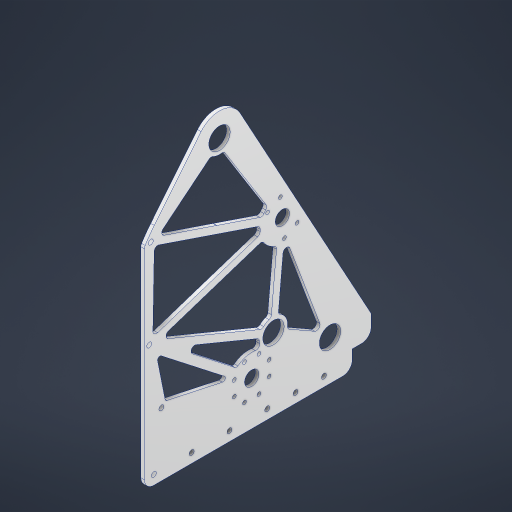
# Autodesk Inventor part: CORL_001_MainPlate
Saved by Autodesk Inventor 2024.2 (Build 282272000, 272)
## iProperties
Created: 2024-08-01
Part Number: CORL_001_MainPlate
Material: Aluminum 6061
Document SubType Name: Modeling
Designer: Bryan
Density: 2.7 g/cm^3
Appearance: Aluminum - Flat
Mass: 689.904 g
Surface Area: 1304.9 cm^2
Volume: 255.52 cm^3
Author: Bryan
Autodesk Inventor part; units mm, degrees
ref_plane "YZ Plane" through (0, 0, 0) normal (1, 0, 0) x (0, 1, 0)
ref_plane "XZ Plane" through (0, 0, 0) normal (0, 1, 0) x (-1, 0, 0)
ref_plane "XY Plane" through (0, 0, 0) normal (0, 0, 1) x (1, 0, 0)
sketch "Sketch1" plane through (0, 0, 0) normal (1, 0, 0) x (0, 1, 0)
  line L0 (0, 0) -> (0, -205.0034) construction
  circle A0 centre (0, 0) radius 25.4 construction
  circle A1 centre (0, -205.0034) radius 25.4 construction
  circle A2 centre (0, 0) radius 14.2875 construction
  circle A3 centre (0, -205.0034) radius 14.2875
  line L1 (0, -266.7) -> (406.4, -266.7) construction
  line L2 (0, 0) -> (0, 69.85) construction
  line L3 (0, 69.85) -> (406.4, 69.85) construction
  line L4 (-25.4, 0) -> (-25.4, -205.0034) construction
  arc A4 (-25.4, 0) -> (-25.4, 0) centre (0, 0) ccw construction
  arc A5 (-25.4, -205.0034) -> (0, -230.4034) centre (0, -205.0034) ccw construction
  line L5 (-53.975, 44.45) -> (-28.575, 44.45)
  line L6 (-28.575, 44.45) -> (-28.575, -234.95) construction
  line L7 (-28.575, -234.95) -> (-53.975, -234.95)
  line L8 (-53.975, -234.95) -> (-53.975, 44.45)
  line L9 (-28.575, -234.95) -> (-28.575, -260.35)
  circle A6 centre (-41.275, 44.45) radius 3.2512 construction
  circle A7 centre (-41.275, 31.75) radius 3.2512
  circle A8 centre (-41.275, 19.05) radius 3.2512 construction
  circle A9 centre (-41.275, 6.35) radius 3.2512 construction
  circle A10 centre (-41.275, -6.35) radius 3.2512 construction
  circle A11 centre (-41.275, -19.05) radius 3.2512
  circle A12 centre (-41.275, -31.75) radius 3.2512 construction
  circle A13 centre (-41.275, -44.45) radius 3.2512 construction
  circle A14 centre (-41.275, -57.15) radius 3.2512 construction
  circle A15 centre (-41.275, -69.85) radius 3.2512
  circle A16 centre (-41.275, -82.55) radius 3.2512 construction
  circle A17 centre (-41.275, -95.25) radius 3.2512 construction
  circle A18 centre (-41.275, -107.95) radius 3.2512 construction
  circle A19 centre (-41.275, -120.65) radius 3.2512
  circle A20 centre (-41.275, -133.35) radius 3.2512 construction
  circle A21 centre (-41.275, -146.05) radius 3.2512 construction
  circle A22 centre (-41.275, -158.75) radius 3.2512
  circle A23 centre (-41.275, -171.45) radius 3.2512 construction
  circle A24 centre (-41.275, -184.15) radius 3.2512 construction
  circle A25 centre (-41.275, -196.85) radius 3.2512
  circle A26 centre (-41.275, -209.55) radius 3.2512 construction
  circle A27 centre (-41.275, -222.25) radius 3.2512 construction
  circle A28 centre (-41.275, -234.95) radius 3.2512 construction
  line L10 (0, -205.0034) -> (142.7545, -151.6469) construction
  circle A29 centre (171.3054, -140.9756) radius 30.48 construction
  circle A30 centre (171.3054, -140.9756) radius 9.525
  circle A31 centre (171.3054, -140.9756) radius 30 construction
  circle A32 centre (155.3994, -160.7786) radius 2.4892
  circle A33 centre (146.0553, -143.7312) radius 2.4892
  circle A34 centre (196.5555, -138.2201) radius 2.4892
  circle A35 centre (187.2114, -121.1727) radius 2.4892
  line L11 (196.5555, -138.2201) -> (187.2114, -121.1727) construction
  line L12 (187.2114, -121.1727) -> (146.0553, -143.7312) construction
  line L13 (146.0553, -143.7312) -> (155.3994, -160.7786) construction
  line L14 (155.3994, -160.7786) -> (196.5555, -138.2201) construction
  circle A36 centre (171.3054, -140.9756) radius 25.4 construction
  line L15 (0, 0) -> (249.8384, -215.9) construction
  circle A37 centre (305.9915, -56.4229) radius 25.4 construction
  arc A38 (305.9915, -56.4229) -> (0, 0) centre (139.099, -103.5757) ccw construction
  line L16 (0, -205.0034) -> (59.0925, -345.4806) construction
  line L17 (59.0925, -345.4806) -> (281.6851, -514.35) construction
  circle A39 centre (281.6851, -514.35) radius 50.8 construction
  line L18 (294.3851, -565.15) -> (268.9851, -565.15) construction
  circle A40 centre (59.0925, -345.4806) radius 50.8 construction
  circle A41 centre (0, -205.0034) radius 152.4 construction
  line L19 (0, -205.0034) -> (152.0099, -215.9) construction
  line L20 (152.0099, -215.9) -> (403.3467, -93.8582) construction
  circle A42 centre (403.3467, -93.8582) radius 50.8 construction
  circle A43 centre (152.0099, -215.9) radius 50.8 construction
  line L21 (305.9915, -56.4229) -> (231.2092, 35.8159) construction
  circle A44 centre (231.2092, 35.8159) radius 6.35 construction
  circle A45 centre (231.2092, 35.8159) radius 3.2512
  circle A46 centre (305.9915, -56.4229) radius 14.2875
  circle A47 centre (403.3467, -93.8582) radius 25.4 construction
  circle A48 centre (152.0099, -215.9) radius 25.4 construction
  line L22 (392.252, -71.0094) -> (140.9152, -193.0512) construction
  line L23 (163.1047, -238.7488) -> (414.4414, -116.707) construction
  circle A49 centre (305.9915, -56.4229) radius 31.75 construction
  circle A50 centre (59.0925, -345.4806) radius 25.4 construction
  line L24 (0, -205.0034) -> (80.5364, -331.8675) construction
  circle A51 centre (112.4851, 38.0456) radius 6.35 construction
  circle A52 centre (112.4851, 38.0456) radius 3.2512
  line L25 (231.2092, 35.8159) -> (112.4851, 38.0456) construction
  line L26 (112.4851, 38.0456) -> (0, 0) construction
  line L27 (-28.575, 44.45) -> (110.7715, 67.5208)
  line L28 (248.2424, 31.1989) -> (325.973, -31.749)
  arc A53 (248.2424, 31.1989) -> (110.7715, 67.5208) centre (139.099, -103.5757) ccw
  line L29 (-28.575, -260.35) -> (0, -260.35)
  arc A54 (321.2522, -84.2648) -> (325.973, -31.749) centre (305.9915, -56.4229) ccw
  line L30 (321.2522, -84.2648) -> (0, -260.35)
  circle A55 centre (4.9608, -99.7986) radius 9.6012
  circle A56 centre (4.9608, -99.7986) radius 25.4 construction
  circle A57 centre (4.9608, -99.7986) radius 30 construction
  circle A58 centre (43.377, -129.0086) radius 14.2875
  circle A59 centre (28.4274, -90.0784) radius 2.4892
  circle A60 centre (14.681, -76.3321) radius 2.4892
  circle A61 centre (-4.7593, -76.3321) radius 2.4892
  circle A62 centre (-18.5057, -90.0784) radius 2.4892
  circle A63 centre (-18.5057, -109.5188) radius 2.4892
  circle A64 centre (-4.7593, -123.2651) radius 2.4892
  circle A65 centre (14.681, -123.2651) radius 2.4892
  circle A66 centre (28.4274, -109.5188) radius 2.4892
  line L31 (-18.5057, -90.0784) -> (-18.5057, -109.5188) construction
  circle A67 centre (43.377, -129.0086) radius 38.1 construction
  circle A68 centre (4.9608, -99.7986) radius 10.16 construction
  point P0 (-41.275, 44.45)
  point P1 (281.6851, -565.15)
  dimension "d165" = 50.8
  dimension "d217" = 50.8
  dimension "d0" = 205.0034
  dimension "d1" = 50.8
  dimension "d3" = 28.575
  dimension "d4" = 28.575
  dimension "d15" = 69.85
  dimension "d19" = 25.4
  dimension "d21" = 3.175
  dimension "d22" = 44.45
  dimension "d23" = 6.5024
  dimension "d27" = 12.7
  dimension "d68" = 60.96
  dimension "d73" = 152.4
  dimension "d74" = 19.05
  dimension "d93" = 60
  dimension "d130" = 4.9784
  dimension "d132" = 50.8
  dimension "d133" = 279.4
  dimension "d139" = 25.4
  dimension "d144" = 6.35
  dimension "d145" = 406.4
  dimension "d147" = 330.2
  dimension "d148" = 50.8
  dimension "d149" = 311.15
  dimension "d151" = 50.8
  dimension "d152" = 279.4
  dimension "d153" = 101.6
  dimension "d154" = 304.8
  dimension "d155" = 150
  dimension "d156" = 150
  dimension "d157" = 12.7
  dimension "d158" = 6.5024
  dimension "d161" = 340.1572
  dimension "d162" = 50.8
  dimension "d163" = 50.8
  dimension "d164" = 63.5
  dimension "d166" = 12.7
  dimension "d167" = 6.5024
  dimension "d168" = 9.594
  dimension "d170" = 24.594
  dimension "d186" = 19.4403
  dimension "d215" = 76.2
  dimension "d216" = 19.2024
  dimension "d218" = 60
  dimension "d219" = 28.575
  dimension "d221" = 4.9784
  dimension "d224" = 360
  dimension "d247" = 87.503
  dimension "d256" = 76.2
  dimension "d257" = 20.32
  dimension "d258" = 304.1396
  dimension "d266" = 29.21
  dimension "d268" = 118.745
  constraints: 66 centre point, 65 end point, 29 coincident, 25 point on circle, 16 tangent, 10 equal radius, 7 equal length, 7 vertical, 6 horizontal, 4 parallel, 4 vertical alignment, 3 midpoint, 1 concentric, 1 perpendicular, 1 point on line, 72 other
  measures "d0" distance of L0.start L0.end
  measures "d1" diameter of A0
  measures "d3" diameter of A2
  measures "d4" diameter of A3
  measures "d15" distance of L2.start L2.end
  measures "d19" distance of L5.start L5.end
  measures "d21" distance between parallel lines of L4 L6
  measures "d22" distance from line of L5 L0.start
  measures "d23" diameter of A6
  measures "d27" distance of A6.centre A7.centre
  measures "d68" diameter of A29
  measures "d73" distance of L0.end L10.end
  measures "d74" diameter of A30
  measures "d93" diameter of A31
  measures "d130" diameter of A32
  measures "d132" diameter of A36
  measures "d133" distance between parallel lines of L5 L7
  measures "d139" distance of L6.end L9.end
  measures "d144" vertical distance of L9.end L1.start
  measures "d145" distance of L2.end L3.end
  measures "d147" distance of L0.start L15.end
  measures "d148" diameter of A37
  measures "d149" distance of L0.start L21.start
  measures "d151" vertical distance of L1.end L15.end
  measures "d152" distance of L16.end L17.end
  measures "d153" diameter of A39
  measures "d154" distance from line of L9.end L18
  measures "d155" angle of L17 L16
  measures "d156" angle of L19 L20
  measures "d157" diameter of A44
  measures "d158" diameter of A45
  measures "d161" distance of L0.end A46.centre
  measures "d162" diameter of A47
  measures "d163" diameter of A48
  measures "d164" diameter of A49
  measures "d166" diameter of A51
  measures "d167" diameter of A52
  measures "d168" angle of L16 L24
  measures "d170" angle of L19 L10
  measures "d186" distance of L12.end L13.end
  measures "d215" distance from line of L21.start L20
  measures "d216" diameter of A55
  measures "d218" diameter of A57
  measures "d219" diameter of A58
  measures "d221" diameter of A59
  measures "d247" distance of L0.end A58.centre
  measures "d256" diameter of A67
  measures "d257" diameter of A68
  measures "d258" distance of A55.centre L21.start
  measures "d266" vertical distance of A55.centre A58.centre
  measures "d268" distance of L25.start L25.end
extrude "Extrusion1" add sketch "Sketch1" along normal blind 4.7625
fillet "Fillet2" radius 12.7 3 edges at (2.3813, -53.975, 44.45) (2.3813, -53.975, -234.95) (2.3813, -28.575, -260.35)
sketch "Sketch5" plane through (4.7625, 0, 0) normal (1, 0, 0) x (0, 0, -1)
  circle A0 centre (-35.8159, 231.2092) radius 6.35
  circle A1 centre (-38.0456, 112.4851) radius 6.35
  line L0 (-38.1, -28.0529) -> (-64.4683, 131.2102)
  arc A2 (-52.8092, 211.4673) -> (-64.4683, 131.2102) centre (117.2224, 145.7909) ccw
  line L1 (-52.8092, 211.4673) -> (36.6838, 321.9767)
  arc A3 (78.6964, 318.2001) -> (36.6838, 321.9767) centre (56.4229, 305.9915) ccw
  line L2 (78.6964, 318.2001) -> (254, -1.6262)
  line L3 (254, -1.6262) -> (254, -15.875)
  arc A4 (247.65, -22.225) -> (254, -15.875) centre (247.65, -15.875) ccw
  line L4 (247.65, -22.225) -> (228.6, -22.225)
  line L5 (228.6, -22.225) -> (228.6, -41.275)
  arc A5 (222.25, -47.625) -> (228.6, -41.275) centre (222.25, -41.275) ccw
  line L6 (222.25, -47.625) -> (-31.75, -47.625)
  arc A6 (-38.1, -41.275) -> (-31.75, -47.625) centre (-31.75, -41.275) ccw
  line L7 (-38.1, -41.275) -> (-38.1, -28.0529)
  circle A7 centre (205.0034, 0) radius 19.05
  circle A8 centre (140.9756, 171.3054) radius 30
  circle A9 centre (56.4229, 305.9915) radius 19.05
  line L8 (56.4229, 305.9915) -> (-35.8159, 231.2092)
  line L9 (-35.8159, 231.2092) -> (-38.0456, 112.4851)
  line L10 (129.0086, 43.377) -> (205.0034, 0)
  line L11 (205.0034, 0) -> (140.9756, 171.3054)
  line L12 (140.9756, 171.3054) -> (56.4229, 305.9915)
  line L13 (-31.0958, 228.9049) -> (55.2471, 298.9071)
  line L14 (55.2471, 298.9071) -> (136.6843, 169.1839)
  line L15 (136.6843, 169.1839) -> (195.9348, 10.66)
  line L16 (195.9348, 10.66) -> (115.3502, 56.6568)
  line L17 (-33.158, 119.104) -> (-31.0958, 228.9049)
  line L18 (-35.8159, 231.2092) -> (140.9756, 171.3054)
  line L19 (140.9756, 171.3054) -> (-38.0456, 112.4851)
  line L20 (-38.0456, 112.4851) -> (129.0086, 43.377)
  line L21 (140.9756, 171.3054) -> (129.0086, 43.377)
  line L22 (-43.616, 109.6356) -> (110.1438, 46.0272)
  line L23 (-37.0067, 117.2093) -> (113.7849, 54.8288)
  line L24 (166.2301, 174.5902) -> (-35.0095, 108.4697)
  line L25 (163.2569, 183.6392) -> (-37.9827, 117.5188)
  line L26 (-39.9815, 227.5922) -> (128.8822, 170.3747)
  line L27 (-36.3152, 236.4069) -> (132.5484, 179.1893)
  line L28 (136.8754, 178.6072) -> (122.5489, 25.4557)
  line L29 (146.1797, 175.8036) -> (133.5494, 40.7852)
  line L30 (-36.9307, 171.8472) -> (51.465, 141.8953)
  line L31 (51.465, 141.8953) -> (52.5799, 201.2573)
  line L32 (-36.9307, 171.8472) -> (52.5799, 201.2573)
  line L33 (47.6922, 194.6384) -> (46.8256, 148.4957)
  line L34 (46.8256, 148.4957) -> (-21.8852, 171.7776)
  line L35 (-21.8852, 171.7776) -> (47.6922, 194.6384)
  line L36 (57.4675, 207.8762) -> (56.1044, 135.2948)
  line L37 (56.1044, 135.2948) -> (-51.9763, 171.9167)
  line L38 (-51.9763, 171.9167) -> (57.4675, 207.8762)
  line L39 (51.465, 141.8953) -> (45.4815, 77.9311)
  line L40 (45.4815, 77.9311) -> (134.9921, 107.3412)
  line L41 (51.465, 141.8953) -> (134.9921, 107.3412)
  line L42 (121.2947, 107.8537) -> (50.9003, 84.7245)
  line L43 (50.9003, 84.7245) -> (55.6059, 135.0283)
  line L44 (55.6059, 135.0283) -> (121.2947, 107.8537)
  line L45 (148.6895, 106.8287) -> (40.0627, 71.1377)
  line L46 (40.0627, 71.1377) -> (47.3241, 148.7623)
  line L47 (47.3241, 148.7623) -> (148.6895, 106.8287)
  line L48 (52.5799, 201.2573) -> (56.4229, 305.9915)
  line L49 (48.055, 207.819) -> (51.2959, 296.1452)
  line L50 (57.4693, 204.629) -> (60.8161, 295.839)
  arc A10 (247.65, -28.575) -> (260.35, -15.875) centre (247.65, -15.875) ccw projected
  line L51 (260.35, -15.875) -> (260.35, 0) projected
  line L52 (260.35, 0) -> (84.2648, 321.2522) projected
  arc A11 (84.2648, 321.2522) -> (31.749, 325.973) centre (56.4229, 305.9915) ccw projected
  line L53 (31.749, 325.973) -> (-31.1989, 248.2424) projected
  arc A12 (-31.1989, 248.2424) -> (-67.5208, 110.7715) centre (103.5757, 139.099) ccw projected
  line L54 (-67.5208, 110.7715) -> (-44.45, -28.575) projected
  line L55 (-44.45, -28.575) -> (-44.45, -41.275) projected
  arc A13 (-44.45, -41.275) -> (-31.75, -53.975) centre (-31.75, -41.275) ccw projected
  line L56 (-31.75, -53.975) -> (222.25, -53.975) projected
  arc A14 (222.25, -53.975) -> (234.95, -41.275) centre (222.25, -41.275) ccw projected
  line L57 (234.95, -41.275) -> (234.95, -28.575) projected
  line L58 (234.95, -28.575) -> (247.65, -28.575) projected
  circle A15 centre (109.5188, 28.4274) radius 2.4892 projected
  circle A16 centre (123.2651, -4.7593) radius 2.4892 projected
  circle A17 centre (90.0784, -18.5057) radius 2.4892 projected
  circle A18 centre (76.3321, 14.681) radius 2.4892 projected
  circle A19 centre (129.0086, 43.377) radius 14.2875 projected
  circle A20 centre (99.7986, 4.9608) radius 9.6012 projected
  circle A21 centre (196.85, -41.275) radius 3.2512 projected
  circle A22 centre (158.75, -41.275) radius 3.2512 projected
  circle A23 centre (120.65, -41.275) radius 3.2512 projected
  circle A24 centre (69.85, -41.275) radius 3.2512 projected
  circle A25 centre (19.05, -41.275) radius 3.2512 projected
  circle A26 centre (-31.75, -41.275) radius 3.2512 projected
  circle A27 centre (90.0784, 28.4274) radius 2.4892 projected
  circle A28 centre (76.3321, -4.7593) radius 2.4892 projected
  circle A29 centre (109.5188, -18.5057) radius 2.4892 projected
  circle A30 centre (123.2651, 14.681) radius 2.4892 projected
  circle A31 centre (-38.0456, 112.4851) radius 3.2512 projected
  circle A32 centre (56.4229, 305.9915) radius 14.2875 projected
  circle A33 centre (-35.8159, 231.2092) radius 3.2512 projected
  circle A34 centre (121.1727, 187.2114) radius 2.4892 projected
  circle A35 centre (138.2201, 196.5555) radius 2.4892 projected
  circle A36 centre (143.7312, 146.0553) radius 2.4892 projected
  circle A37 centre (160.7786, 155.3994) radius 2.4892 projected
  circle A38 centre (140.9756, 171.3054) radius 9.525 projected
  circle A39 centre (205.0034, 0) radius 14.2875 projected
  circle A40 centre (129.0086, 43.377) radius 19.05
  circle A41 centre (99.7986, 4.9608) radius 30
  line L59 (-38.0456, 112.4851) -> (99.7986, 4.9608)
  line L60 (99.7986, 4.9608) -> (129.0086, 43.377)
  line L61 (-7.4906, 94.691) -> (111.2202, 2.0915)
  line L62 (99.7986, 4.9608) -> (45.4815, 77.9311)
  line L63 (97.3778, 0.237) -> (42.4462, 74.0328)
  line L64 (105.0184, 5.9245) -> (57.8018, 69.3557)
  circle A42 centre (205.0034, 0) radius 14.2875 projected
  line L65 (96.0075, 7.8434) -> (125.2175, 46.2596)
  line L66 (99.7986, 4.9608) -> (205.0034, 0)
  line L67 (100.0229, 9.718) -> (202.5451, 4.8837)
  line L68 (103.5897, 2.0783) -> (132.7997, 40.4945)
  line L69 (126.6477, 39.2409) -> (214.072, -10.66)
  line L70 (214.072, -10.66) -> (145.4367, 172.9728)
  point P0 (0, 0)
  point P1 (142.9587, 141.371)
  point P2 (191.345, 13.2798)
  point P3 (194.0846, 15.6103)
  point P4 (146.8846, 141.8931)
  point P5 (133.4751, 142.2582)
  point P6 (114.3227, 157.5352)
  point P7 (-24.3482, 111.9726)
  point P8 (111.3944, 176.3002)
  point P9 (-31.1765, 224.6087)
  point P10 (-54.5444, 120.5889)
  point P11 (111.3495, 166.5842)
  point P12 (-26.1084, 232.9484)
  point P13 (114.4511, 185.3214)
  point P14 (121.1937, 193.8592)
  point P15 (62.1964, 287.8374)
  point P16 (45.0944, 290.6759)
  point P17 (-32.0431, 178.4661)
  point P18 (37.5344, 201.3268)
  point P19 (36.4195, 141.9648)
  point P20 (-32.2914, 165.2467)
  point P21 (57.2193, 194.6568)
  point P22 (56.3527, 148.5142)
  point P23 (41.3406, 84.7981)
  point P24 (46.0462, 135.1019)
  point P25 (129.5733, 100.5478)
  point P26 (59.1789, 77.4186)
  point P27 (65.1624, 141.3828)
  point P28 (130.8512, 114.2082)
  point P29 (57.5899, 207.9164)
  point P30 (60.5058, 287.3842)
  point P31 (62.7917, 204.659)
  point P32 (53.8187, 207.9057)
  point P33 (50.9872, 287.7334)
  point P34 (129.8235, 180.1127)
  point P35 (60.6149, 290.3566)
  point P36 (51.6549, 146.9706)
  point P37 (51.5611, 147.0095)
  point P38 (51.5598, 146.9394)
  point P39 (52.6031, 206.2779)
  point P40 (57.407, 204.6502)
  point P41 (143.7837, 150.1896)
  point P42 (134.0364, 45.9909)
  point P43 (63.2565, 21.7112)
  point P44 (234.95, -34.925)
  point P45 (125.5214, 57.2324)
  point P46 (57.3578, 26.3886)
  point P47 (53.4598, 29.4795)
  point P48 (125.9847, 62.1855)
  point P49 (119.6707, 54.1907)
  point P50 (135.005, 56.3453)
  point P51 (135.4683, 61.2984)
  point P52 (96.5825, 26.6734)
  point P53 (88.0937, 51.1529)
  point P54 (147.3887, 38.3696)
  point P55 (59.6038, 66.9349)
  point P56 (85.9328, 31.5642)
  point P57 (78.2922, 25.8768)
  point P58 (30.2452, 75.5228)
  point P59 (-48.3709, 98.4476)
  point P60 (79.3732, 26.9336)
  point P61 (43.7757, 136.1322)
  point P62 (43.3258, 136.249)
  point P63 (140.0614, 110.3981)
  point P64 (139.4433, 103.7907)
  point P65 (145.8295, 144.7161)
  point P66 (144.4367, 148.4424)
  point P67 (195.8262, 10.9504)
  point P68 (195.6655, 10.8137)
  point P69 (143.0683, 40.8356)
  point P70 (133.7051, 173.9295)
  point P71 (-37.0246, 166.8505)
  point P72 (-37.9264, 118.834)
  point P73 (-35.5419, 118.3207)
  point P74 (132.5563, 175.7595)
  point P75 (131.6523, 173.2551)
  point P76 (59.5514, 292.0507)
  point P77 (48.9587, 293.8088)
  point P78 (74.9197, 30.4075)
  point P79 (114.373, 31.1827)
  point P80 (121.1704, 26.0143)
  point P81 (52.7661, 206.3315)
  point P82 (52.7621, 206.224)
  point P83 (55.7244, 286.9543)
  point P84 (-31.4417, 234.7555)
  point P85 (41.6252, 293.9943)
  point P86 (-36.836, 176.8913)
  point P87 (-35.8769, 227.9586)
  point P88 (-33.2904, 233.2567)
  point P89 (-23.9775, 101.5114)
  point P90 (76.144, 23.4124)
  dimension "d191" = 12.7
  dimension "d192" = 60
  dimension "d193" = 4.7625
  dimension "d194" = 4.7625
  dimension "d195" = 4.7625
  dimension "d196" = 4.7625
  dimension "d197" = 4.7625
  dimension "d198" = 4.7625
  dimension "d199" = 4.7625
  dimension "d200" = 4.7625
  dimension "d201" = 4.7625
  dimension "d204" = 4.7625
  dimension "d205" = 4.7625
  dimension "d206" = 4.7625
  dimension "d207" = 4.7625
  dimension "d210" = 4.7625
  dimension "d211" = 4.7625
  dimension "d226" = 4.7625
  dimension "d227" = 6.35
  dimension "d228" = 6.35
  dimension "d229" = 6.35
  dimension "d230" = 6.35
  dimension "d231" = 6.35
  dimension "d232" = 6.35
  dimension "d233" = 6.35
  dimension "d234" = 19.05
  dimension "d235" = 6.35
  dimension "d236" = 6.35
  dimension "d237" = 6.35
  dimension "d238" = 4.7625
  dimension "d239" = 4.7625
  dimension "d240" = 4.7625
  dimension "d242" = 6.35
  dimension "d243" = 6.35
  dimension "d244" = 6.35
  dimension "d248" = 4.7625
  dimension "d249" = 60
  dimension "d250" = 4.7625
  dimension "d251" = 4.7625
  dimension "d252" = 4.7625
  dimension "d259" = 4.7625
  dimension "d260" = 4.7625
  dimension "d261" = 4.7625
  dimension "d262" = 4.7625
  constraints: 126 end point, 15 parallel, 14 point on circle, 12 centre point, 8 point on line, 6 midpoint, 5 coincident, 2 concentric, 1 equal radius, 11 other
  measures "d191" diameter of A0
  measures "d192" diameter of A8
  measures "d193" distance between parallel lines of L8 L13
  measures "d194" distance between parallel lines of L20 L22
  measures "d195" distance between parallel lines of L20 L23
  measures "d196" distance between parallel lines of L19 L24
  measures "d197" distance between parallel lines of L19 L25
  measures "d198" distance between parallel lines of L18 L26
  measures "d199" distance between parallel lines of L18 L27
  measures "d200" distance between parallel lines of L21 L28
  measures "d201" distance between parallel lines of L21 L29
  measures "d204" distance between parallel lines of L32 L35
  measures "d205" distance between parallel lines of L32 L38
  measures "d206" distance between parallel lines of L41 L44
  measures "d207" distance between parallel lines of L41 L47
  measures "d210" distance between parallel lines of L48 L49
  measures "d211" distance between parallel lines of L48 L50
  measures "d226" distance between parallel lines of L17 L9
  measures "d228" distance between parallel lines of L56 L6
  measures "d229" distance between parallel lines of L52 L2
  measures "d230" distance from line of point (234.95, -34.925) L5
  measures "d231" distance between parallel lines of L58 L4
  measures "d232" distance between parallel lines of L51 L3
  measures "d233" radius of A4
  measures "d234" distance of L4.end L5.end
  measures "d235" radius of A5
  measures "d236" radial gap between concentric circles of A11 A3
  measures "d237" distance between parallel lines of L53 L1
  measures "d238" radial gap between concentric circles of A9 A32
  measures "d239" radial gap between concentric circles of A39 A7
  measures "d240" radial gap between concentric circles of A19 A40
  measures "d242" distance between parallel lines of L54 L0
  measures "d243" distance between parallel lines of L55 L7
  measures "d244" radius of A6
  measures "d248" distance between parallel lines of L10 L16
  measures "d249" diameter of A41
  measures "d250" distance between parallel lines of L59 L61
  measures "d251" distance between parallel lines of L62 L63
  measures "d252" distance between parallel lines of L62 L64
  measures "d259" distance between parallel lines of L60 L65
  measures "d260" distance between parallel lines of L66 L67
  measures "d261" distance between parallel lines of L60 L68
  measures "d262" distance between parallel lines of L10 L69
extrude "Extrusion5" cut sketch "Sketch5" against normal blind 4.7625 contours L13 A9 L49 L27 | L8 L9 A33 L1 | L49 A9 L48 L38 L27 | L1 A33 | L26 L38 L17 | L26 L32 L17 L38 | A9 L50 L27 L36 L38 L48 | L48 L38 L36 L27 | L31 L47 L46 L25 L30 L17 L32 L26 | L26 L36 L25 L47 L31 | L14 A8 L27 L50 A9 | L26 A8 L25 L36 | L47 L25 L31 | L31 L25 L46 L47 | L30 L25 L37 L17 | L37 L25 L17 | A8 L28 L47 L24 | L47 L28 L41 L24 | L37 L36 L24 L41 L28 L40 L23 L39 | L24 L36 L37 | L39 L23 L46 L24 | L46 L23 L24 | L15 A7 L16 A40 L29 L45 L47 A8 | L22 L46 L45 L63 L61 | L40 L28 L45 L23 | L22 L63 L45 L46 | L63 L45 L22 L62 A41 L61 | L47 L45 L29 | L45 L28 A40 L23 | L22 L45 L63 | L22 L64 A41 L62 | A19 L16 L28 L20 | L20 L28 L65 A19 | A40 L65 A41 L64 L22 | A19 L10 L29 L16 | L28 L16 L21 L20 | L20 L65 L28 | L65 L28 L60 A19 | A40 A41 L65 | L16 L29 L10 L21 | A19 L69 L68 L28 L60 L10 | A19 L68 L69 | L20 L60 L28 L65 | L60 L28 A19 | L33 L34 L35 | L42 L43 L44
fillet "Fillet5" radius 4.7625 23 edges at (2.3813, 224.6087, 31.1765) (2.3813, 232.9484, 26.1084) (2.3813, 290.6759, -45.0944) (2.3813, 287.8374, -62.1964) (2.3813, 193.8592, -121.1937) (2.3813, 185.3214, -114.4511) (2.3813, 176.3002, -111.3944) (2.3813, 166.5842, -111.3495) (2.3813, 157.5352, -114.3227) (2.3813, 142.2582, -133.4751) (2.3813, 141.371, -142.9587) (2.3813, 141.8931, -146.8846) (2.3813, 111.9726, 24.3482) (2.3813, 46.0272, -110.1438) (2.3813, 54.8288, -113.7849) (2.3813, 62.1855, -125.9847) (2.3813, 61.2984, -135.4683) (2.3813, 38.3696, -147.3887) (2.3813, 15.6103, -194.0846) (2.3813, 13.2798, -191.345) (2.3813, 119.104, 33.158) (2.3813, 94.691, 7.4906) (2.3813, 31.1827, -114.373)
sketch "Sketch6" plane through (4.7625, 0, 0) normal (1, 0, 0) x (0, 0, -1)
  circle A0 centre (-38.0456, 112.4851) radius 3.2512 construction
  circle A1 centre (-31.75, -41.275) radius 3.2512 construction
  line L0 (-38.0456, 112.4851) -> (-31.75, -41.275) construction
  circle A2 centre (19.05, -41.275) radius 3.2512 construction
  arc A3 (-38.0456, 112.4851) -> (19.05, -41.275) centre (226.7387, 123.3266) ccw construction
  circle A4 centre (-21.6928, 31.0767) radius 3.2512
  point P0 (0, 0)
  dimension "d263" = 6.5024
  constraints: 3 point on circle, 2 centre point, 2 end point, 1 tangent
  measures "d263" diameter of A4
extrude "Extrusion6" cut sketch "Sketch6" against normal blind 4.7625
sketch "Sketch8" plane through (4.7625, 0, 0) normal (1, 0, 0) x (0, 0, -1)
  circle A0 centre (-21.6928, 31.0767) radius 3.2512 projected
  circle A1 centre (-21.6928, 31.0767) radius 6.35
  circle A2 centre (-38.0456, 112.4851) radius 3.2512 projected
  circle A3 centre (-38.0456, 112.4851) radius 6.35
  circle A4 centre (99.7986, 4.9608) radius 9.6012 projected
  circle A5 centre (99.7986, 4.9608) radius 30
  circle A6 centre (-21.6928, 31.0767) radius 3.2512 projected
  arc A7 (104.7687, 34.5463) -> (79.3732, 26.9336) centre (99.7986, 4.9608) ccw projected
  line L0 (24.8849, 81.2977) -> (107.0211, 47.319) projected
  arc A8 (109.9621, 43.01) -> (107.0211, 47.319) centre (105.2005, 42.9182) ccw projected
  arc A9 (109.9621, 43.01) -> (110.2479, 40.0698) centre (129.0086, 43.377) ccw projected
  arc A10 (104.7687, 34.5463) -> (110.2479, 40.0698) centre (105.5577, 39.243) ccw projected
  line L1 (110.6622, 56.1206) -> (-12.4714, 107.0594) projected
  arc A11 (-12.1375, 115.9847) -> (-12.4714, 107.0594) centre (-10.6508, 111.4602) ccw projected
  line L2 (-12.1375, 115.9847) -> (110.7006, 156.3451) projected
  arc A12 (116.1313, 154.49) -> (110.7006, 156.3451) centre (112.1872, 151.8206) ccw projected
  arc A13 (116.1313, 154.49) -> (130.1041, 143.3445) centre (140.9756, 171.3054) ccw projected
  arc A14 (133.12, 138.4622) -> (130.1041, 143.3445) centre (128.3782, 138.9058) ccw projected
  line L3 (133.12, 138.4622) -> (126.2995, 65.5502) projected
  arc A15 (123.0479, 61.4705) -> (126.2995, 65.5502) centre (121.5577, 65.9938) ccw projected
  arc A16 (123.0479, 61.4705) -> (115.7879, 57.0925) centre (129.0086, 43.377) ccw projected
  arc A17 (110.6622, 56.1206) -> (115.7879, 57.0925) centre (112.4827, 60.5214) ccw projected
  arc A18 (184.5053, 17.1838) -> (191.3273, 22.9873) centre (186.8662, 21.3199) ccw projected
  line L4 (184.5053, 17.1838) -> (150.3237, 36.6943) projected
  arc A19 (147.9494, 41.3398) -> (150.3237, 36.6943) centre (152.6845, 40.8305) ccw projected
  arc A20 (147.9494, 41.3398) -> (138.2216, 60.051) centre (129.0086, 43.377) ccw projected
  arc A21 (135.7831, 64.6631) -> (138.2216, 60.051) centre (140.5249, 64.2195) ccw projected
  line L5 (135.7831, 64.6631) -> (141.8499, 129.5174) projected
  arc A22 (151.0528, 130.7413) -> (141.8499, 129.5174) centre (146.5917, 129.0739) ccw projected
  line L6 (151.0528, 130.7413) -> (191.3273, 22.9873) projected
  arc A23 (111.0119, 172.7792) -> (110.9995, 170.1087) centre (140.9756, 171.3054) ccw projected
  arc A24 (107.7274, 165.3942) -> (110.9995, 170.1087) centre (106.2408, 169.9187) ccw projected
  line L7 (107.7274, 165.3942) -> (-26.7837, 121.1984) projected
  arc A25 (-33.032, 125.8124) -> (-26.7837, 121.1984) centre (-28.2703, 125.7229) ccw projected
  line L8 (-33.032, 125.8124) -> (-31.2988, 218.0977) projected
  arc A26 (-25.0087, 222.5189) -> (-31.2988, 218.0977) centre (-26.5371, 218.0083) ccw projected
  line L9 (-25.0087, 222.5189) -> (107.7835, 177.5237) projected
  arc A27 (111.0119, 172.7792) -> (107.7835, 177.5237) centre (106.2551, 173.0131) ccw projected
  line L10 (-19.4002, 238.387) -> (42.4693, 288.5476) projected
  arc A28 (47.6595, 289.0768) -> (42.4693, 288.5476) centre (45.4686, 284.8482) ccw projected
  arc A29 (47.6595, 289.0768) -> (59.2523, 287.1528) centre (56.4229, 305.9915) ccw projected
  arc A30 (63.9932, 284.9753) -> (59.2523, 287.1528) centre (59.9596, 282.4431) ccw projected
  line L11 (63.9932, 284.9753) -> (119.1666, 197.0882) projected
  arc A31 (118.6735, 191.3707) -> (119.1666, 197.0882) centre (115.1331, 194.556) ccw projected
  arc A32 (118.6735, 191.3707) -> (116.2878, 188.3497) centre (140.9756, 171.3054) ccw projected
  arc A33 (110.8402, 186.5449) -> (116.2878, 188.3497) centre (112.3686, 191.0555) ccw projected
  line L12 (110.8402, 186.5449) -> (52.7621, 206.224) projected
  line L13 (52.7621, 206.224) -> (52.7661, 206.3315) projected
  line L14 (52.7661, 206.3315) -> (52.6031, 206.2779) projected
  line L15 (52.6031, 206.2779) -> (-17.9293, 230.177) projected
  arc A34 (-19.4002, 238.387) -> (-17.9293, 230.177) centre (-16.401, 234.6876) ccw projected
  arc A35 (247.65, -28.575) -> (260.35, -15.875) centre (247.65, -15.875) ccw projected
  line L16 (260.35, -15.875) -> (260.35, 0) projected
  line L17 (260.35, 0) -> (84.2648, 321.2522) projected
  arc A36 (84.2648, 321.2522) -> (31.749, 325.973) centre (56.4229, 305.9915) ccw projected
  line L18 (31.749, 325.973) -> (-31.1989, 248.2424) projected
  arc A37 (-31.1989, 248.2424) -> (-67.5208, 110.7715) centre (103.5757, 139.099) ccw projected
  line L19 (-67.5208, 110.7715) -> (-44.45, -28.575) projected
  line L20 (-44.45, -28.575) -> (-44.45, -41.275) projected
  arc A38 (-44.45, -41.275) -> (-31.75, -53.975) centre (-31.75, -41.275) ccw projected
  line L21 (-31.75, -53.975) -> (222.25, -53.975) projected
  arc A39 (222.25, -53.975) -> (234.95, -41.275) centre (222.25, -41.275) ccw projected
  line L22 (234.95, -41.275) -> (234.95, -28.575) projected
  line L23 (234.95, -28.575) -> (247.65, -28.575) projected
  circle A40 centre (109.5188, 28.4274) radius 2.4892 projected
  circle A41 centre (123.2651, -4.7593) radius 2.4892 projected
  circle A42 centre (90.0784, -18.5057) radius 2.4892 projected
  circle A43 centre (76.3321, 14.681) radius 2.4892 projected
  circle A44 centre (129.0086, 43.377) radius 14.2875 projected
  circle A45 centre (99.7986, 4.9608) radius 9.6012 projected
  circle A46 centre (196.85, -41.275) radius 3.2512 projected
  circle A47 centre (158.75, -41.275) radius 3.2512 projected
  circle A48 centre (120.65, -41.275) radius 3.2512 projected
  circle A49 centre (69.85, -41.275) radius 3.2512 projected
  circle A50 centre (19.05, -41.275) radius 3.2512 projected
  circle A51 centre (-31.75, -41.275) radius 3.2512 projected
  circle A52 centre (90.0784, 28.4274) radius 2.4892 projected
  circle A53 centre (76.3321, -4.7593) radius 2.4892 projected
  circle A54 centre (109.5188, -18.5057) radius 2.4892 projected
  circle A55 centre (123.2651, 14.681) radius 2.4892 projected
  circle A56 centre (-38.0456, 112.4851) radius 3.2512 projected
  circle A57 centre (56.4229, 305.9915) radius 14.2875 projected
  circle A58 centre (-35.8159, 231.2092) radius 3.2512 projected
  circle A59 centre (121.1727, 187.2114) radius 2.4892 projected
  circle A60 centre (138.2201, 196.5555) radius 2.4892 projected
  circle A61 centre (143.7312, 146.0553) radius 2.4892 projected
  circle A62 centre (160.7786, 155.3994) radius 2.4892 projected
  circle A63 centre (140.9756, 171.3054) radius 9.525 projected
  circle A64 centre (205.0034, 0) radius 14.2875 projected
  line L24 (-38.0456, 112.4851) -> (-21.6928, 31.0767)
  line L25 (-21.6928, 31.0767) -> (99.7986, 4.9608)
  line L26 (99.7986, 4.9608) -> (-38.0456, 112.4851)
  line L27 (-16.2873, 36.4098) -> (-28.4471, 96.9445)
  line L28 (-28.4471, 96.9445) -> (74.0528, 16.9902)
  line L29 (74.0528, 16.9902) -> (-16.2873, 36.4098)
  line L30 (-44.45, 229.4587) -> (-44.45, -28.575)
  line L31 (79.3732, 26.9336) -> (20.1352, 73.1417) projected
  arc A65 (24.8849, 81.2977) -> (20.1352, 73.1417) centre (23.0644, 76.8969) ccw projected
  point P0 (0, 0)
  point P1 (72.4677, 17.331)
  point P2 (72.7744, 17.9874)
  dimension "d269" = 12.7
  dimension "d270" = 12.7
  dimension "d271" = 60
  dimension "d272" = 6.35
  constraints: 14 end point, 3 centre point, 3 coincident, 1 point on circle, 1 vertical, 2 other
  measures "d269" diameter of A1
  measures "d270" diameter of A3
  measures "d271" diameter of A5
  measures "d272" distance between parallel lines of L24 L27
extrude "Extrusion7" cut sketch "Sketch8" against normal blind 4.7625 contours L29 L27 L28 A5 | L30 L19 A37
fillet "Fillet8" radius 3.175 5 edges at (2.3813, 96.9445, 28.4471) (2.3813, 17.331, -72.4677) (2.3813, 17.9874, -72.7744) (2.3813, 36.4098, 16.2873) (2.3813, 26.9336, -79.3732)
fillet "Fillet9" radius 6.35 1 edges at (2.3813, 229.4587, 44.45)
body "Solid1"
